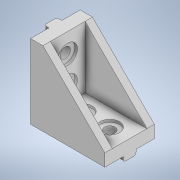
# Autodesk Inventor part: right_angle_profile_mount
Saved by Autodesk Inventor 2021 (Build 250183000, 183)
## iProperties
Created: 2021-02-05
Part Number: right_angle_profile_mount
Material: 일반
Document SubType Name: Modeling
Designer: jun85
Density: 1 g/cm^3
Appearance: 기본값
Author: jun85
Autodesk Inventor part; units mm, degrees
ref_plane "YZ Plane" through (0, 0, 0) normal (1, 0, 0) x (0, 1, 0)
sketch "스케치1" plane through (0, 0, 0) normal (0, 0, 1) x (1, 0, 0)
  line L0 (0, 0) -> (0, 30)
  line L1 (0, 30) -> (5, 30)
  line L2 (5, 30) -> (30, 5)
  line L3 (30, 5) -> (30, 0)
  line L4 (30, 0) -> (0, 0)
  dimension "d0" = 30
  dimension "d1" = 5
  constraints: 10 end point, 4 perpendicular, 1 parallel, 1 vertical
  measures "d0" distance of L0.start L0.end
  measures "d1" distance of L0.end L1.end
extrude "돌출1" add sketch "스케치1" along normal blind 20
sketch "스케치2" plane through (0, 0, 0) normal (-1, 0, 0) x (0, 0, 1)
  line L0 (0, 30) -> (0, 0) projected
  line L1 (0, 0) -> (20, 0) projected
  line L2 (20, 30) -> (20, 0) projected
  line L3 (0, 30) -> (20, 30) projected
  line L4 (0, 30) -> (20, 30) projected
  line L5 (7.4, 30) -> (12.6, 30)
  line L6 (12.6, 30) -> (12.6, 0)
  line L7 (12.6, 0) -> (7.4, 0)
  line L8 (7.4, 0) -> (7.4, 30)
  line L9 (0, 0) -> (20, 30) construction
  line L10 (20, 0) -> (20, 5) projected
  line L11 (0, 5) -> (0, 30) projected
  line L12 (20, 0) -> (0, 30) construction
  line L13 (7.4, 0) -> (12.6, 30) construction
  line L14 (7.4, 30) -> (12.6, 0) construction
  point P0 (10, 15)
  dimension "d4" = 5.2
  constraints: 16 end point, 2 midpoint, 2 parallel, 2 point on line, 1 horizontal, 1 perpendicular
  measures "d4" distance between parallel lines of L6 L8
extrude "돌출2" add sketch "스케치2" along normal blind 2 contours L3 L6 L1 L8
ref_plane "작업 평면1" through (0, 0, 20) normal (-0.7071068, 0.7071068, 0) x (0, 0, -1)
mirror "미러1" about plane through (0, 0, 20) normal (-0.7071068, 0.7071068, 0) of "돌출2"
sketch "스케치3" plane through (0, -2, 7.4) normal (-1, 0, 0) x (0, 0, 1)
  line L0 (0, 2) -> (5.2, 2) projected
  line L1 (0, 2) -> (0, 0) projected
  line L2 (0, 0) -> (5.2, 0) projected
  line L3 (5.2, 2) -> (5.2, 0) projected
  point P0 (-7.4, 2)
extrude "돌출3" add sketch "스케치3" along normal blind 2
fillet "모깎기1" radius 1 4 edges at (-2, 14, 12.6) (14, -2, 12.6) (14, -2, 7.4) (-2, 14, 7.4)
sketch "스케치4" plane through (0, 0, 20) normal (-1, 0, 0) x (0, 0, 1)
  line L0 (-20, 30) -> (0, 30) projected
  line L1 (-7.4, 0) -> (0, 0) projected
  line L2 (-20, 30) -> (0, 0) construction
  line L3 (-20, 0) -> (-20, 5) projected
  line L4 (0, 30) -> (-20, 0) construction
  circle A0 centre (-10, 22) radius 2.1
  circle A1 centre (-10, 11) radius 2.1
  line L5 (-13.5, 25.5) -> (-6.5, 25.5)
  line L6 (-6.5, 25.5) -> (-6.5, 18.5)
  line L7 (-6.5, 18.5) -> (-13.5, 18.5)
  line L8 (-13.5, 18.5) -> (-13.5, 25.5)
  line L9 (-13.5, 25.5) -> (-6.5, 18.5) construction
  line L10 (-6.5, 25.5) -> (-13.5, 18.5) construction
  line L11 (-13.5, 14.5) -> (-6.5, 14.5)
  line L12 (-6.5, 14.5) -> (-6.5, 7.5)
  line L13 (-6.5, 7.5) -> (-13.5, 7.5)
  line L14 (-13.5, 7.5) -> (-13.5, 14.5)
  line L15 (-13.5, 14.5) -> (-6.5, 7.5) construction
  line L16 (-6.5, 14.5) -> (-13.5, 7.5) construction
  point P0 (-10, 15)
  point P1 (-10, 15)
  dimension "d10" = 7
  dimension "d11" = 4
  dimension "d13" = 4.2
  dimension "d16" = 7
  dimension "d17" = 7
  constraints: 28 end point, 6 midpoint, 4 parallel, 2 centre point, 2 equal length, 2 horizontal, 2 perpendicular, 1 equal radius
  measures "d10" distance of point (-10, 15) A0.centre
  measures "d11" distance of point (-10, 15) A1.centre
  measures "d13" diameter of A0
  measures "d16" distance of L5.end L6.end
  measures "d17" distance of L6.end L7.end
extrude "돌출4" cut sketch "스케치4" along normal blind 2 contours A0 | A1 | L5 L6 L7 L8 | L11 L12 L13 L14
extrude "돌출5" cut sketch "스케치4" against normal through all contours A0 | A1
ref_plane "작업 평면2" through (5, 0, 0) normal (-1, 0, 0) x (0, 0, 1)
sketch "스케치5" plane through (5, 0, 0) normal (-1, 0, 0) x (0, 0, 1)
  circle A0 centre (10, 11) radius 2.1 projected
  circle A1 centre (10, 22) radius 2.1 projected
  line L0 (0, 5) -> (0, 30) projected
  line L1 (0, 30) -> (20, 30) projected
  line L2 (20, 5) -> (20, 30) projected
  line L3 (0, 5) -> (20, 5) projected
  line L4 (0, 30) -> (7.4, 30) projected
  line L5 (3, 30) -> (17, 30)
  line L6 (17, 30) -> (17, 5)
  line L7 (17, 5) -> (3, 5)
  line L8 (3, 5) -> (3, 30)
  point P0 (0, 0)
  dimension "d21" = 3
  dimension "d22" = 3
  constraints: 8 end point, 2 parallel, 2 point on line, 1 horizontal, 1 perpendicular
  measures "d21" distance between parallel lines of L0 L8
  measures "d22" distance between parallel lines of L2 L6
extrude "돌출6" cut sketch "스케치5" against normal through all contours L8 L1 L6 L3
mirror "미러2" about plane through (0, 0, 20) normal (-0.7071068, 0.7071068, 0) of "돌출6", "돌출5", "돌출4"
sketch "스케치6" plane through (5, 0, 0) normal (1, 0, 0) x (0, 0, -1)
  line L0 (-3, 5) -> (-17, 5) projected
  line L1 (-3, 30) -> (-3, 5) projected
  line L2 (-3, 30) -> (-17, 30) projected
  line L3 (-17, 5) -> (-17, 30) projected
  circle A0 centre (-10, 11) radius 2.1 projected
  circle A1 centre (-10, 22) radius 2.1 projected
  circle A2 centre (-10, 11) radius 3.9
  circle A3 centre (-10, 22) radius 3.9
  point P0 (0, 0)
  dimension "d25" = 7.8
  constraints: 2 centre point, 2 coincident, 1 equal radius
  measures "d25" diameter of A3
extrude "돌출7" cut sketch "스케치6" against normal blind 1 contours A0 | A1 | A2 | A3
mirror "미러3" about plane through (0, 0, 20) normal (-0.7071068, 0.7071068, 0) of "돌출7"
